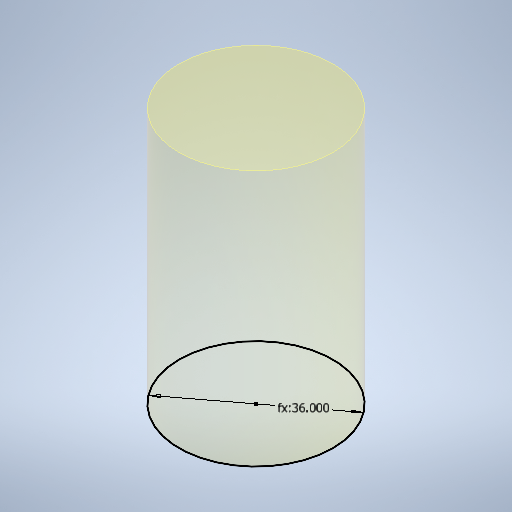
# Autodesk Inventor part: Cylinder-sizing (plug-demo)
Saved by Autodesk Inventor 2026.1 (Build 301233020, 233B)
## iProperties
RuleStatus: InUse
Created: 2025-11-10
Part Number: Cylinder-sizing (plug-demo)
Material: Generic
Document SubType Name: Modeling
Designer: holy
Density: 1 g/cm^3
Appearance: Default
Author: holy
Autodesk Inventor part; units mm, degrees
ref_plane "YZ Plane" through (0, 0, 0) normal (1, 0, 0) x (0, 1, 0)
ref_plane "XZ Plane" through (0, 0, 0) normal (0, 1, 0) x (-1, 0, 0)
ref_plane "XY Plane" through (0, 0, 0) normal (0, 0, 1) x (1, 0, 0)
sketch "Sketch2" plane through (0, 0, 0) normal (0, 1, 0) x (-1, 0, 0)
  circle A0 centre (0, 0) radius 457.2
  dimension "d4" = 914.4
  constraints: 1 centre point, 1 coincident
  measures "d4" diameter of A0
extrude "Extrusion2" add sketch "Sketch2" along normal blind 1524
equation "\"d4\" = Diameter"
equation "\"d5\" = Height"
equation "\"Diameter\" = 914.4"
equation "\"Height\" = 1524"
body "Solid2"
